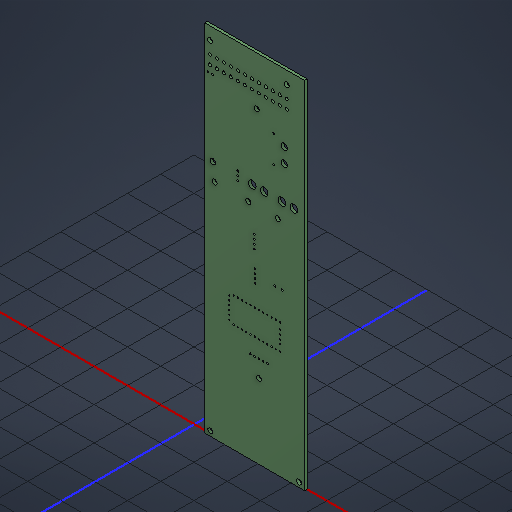
# Autodesk Inventor part: Omnibot_battery_module.brdКонтур
Saved by Autodesk Inventor 2025 (Build 290162000, 162)
## iProperties
Created: 2024-08-15
Part Number: Omnibot_battery_module.brdКонтур
Material: Типовые
Document SubType Name: Modeling
Designer: IvanPetrov
Density: 1 g/cm^3
Appearance: Контур панели
Author: IvanPetrov
Autodesk Inventor part; units mm, degrees
ref_plane "YZ Plane" through (0, 0, 0) normal (1, 0, 0) x (0, 1, 0)
ref_plane "XZ Plane" through (0, 0, 0) normal (0, 1, 0) x (-1, 0, 0)
ref_plane "XY Plane" through (0, 0, 0) normal (0, 0, 1) x (1, 0, 0)
sketch "Эскиз1" plane through (0, 0, 0) normal (0, 0, 1) x (1, 0, 0)
  line L0 (68.1, 149.83) -> (68.1, -63.84)
  line L1 (68.1, -63.84) -> (8.1, -63.84)
  line L2 (8.1, -63.84) -> (8.1, 149.83)
  line L3 (8.1, 149.83) -> (68.1, 149.83)
  circle A0 centre (38.35, 29.21) radius 0.51
  circle A1 centre (38.35, 31.75) radius 0.51
  circle A2 centre (38.35, 34.29) radius 0.51
  circle A3 centre (38.35, 36.83) radius 0.51
  circle A4 centre (37.85, 54.61) radius 0.51
  circle A5 centre (37.85, 52.07) radius 0.51
  circle A6 centre (37.85, 49.53) radius 0.51
  circle A7 centre (37.85, 46.99) radius 0.51
  circle A8 centre (43.86, 79.88) radius 2.275
  circle A9 centre (36.66, 79.88) radius 2.275
  circle A10 centre (61.64, 79.88) radius 2.275
  circle A11 centre (54.44, 79.88) radius 2.275
  circle A12 centre (55.88, 100.33) radius 1.905
  circle A13 centre (55.88, 109.22) radius 1.905
  circle A14 centre (11.19, 134.94) radius 0.9
  circle A15 centre (15.39, 134.94) radius 0.9
  circle A16 centre (19.59, 134.94) radius 0.9
  circle A17 centre (23.79, 134.94) radius 0.9
  circle A18 centre (27.99, 134.94) radius 0.9
  circle A19 centre (32.19, 134.94) radius 0.9
  circle A20 centre (36.39, 134.94) radius 0.9
  circle A21 centre (40.59, 134.94) radius 0.9
  circle A22 centre (44.79, 134.94) radius 0.9
  circle A23 centre (48.99, 134.94) radius 0.9
  circle A24 centre (53.19, 134.94) radius 0.9
  circle A25 centre (57.39, 134.94) radius 0.9
  circle A26 centre (11.19, 129.44) radius 0.9
  circle A27 centre (15.39, 129.44) radius 0.9
  circle A28 centre (19.59, 129.44) radius 0.9
  circle A29 centre (23.79, 129.44) radius 0.9
  circle A30 centre (27.99, 129.44) radius 0.9
  circle A31 centre (32.19, 129.44) radius 0.9
  circle A32 centre (36.39, 129.44) radius 0.9
  circle A33 centre (40.59, 129.44) radius 0.9
  circle A34 centre (44.79, 129.44) radius 0.9
  circle A35 centre (48.99, 129.44) radius 0.9
  circle A36 centre (53.19, 129.44) radius 0.9
  circle A37 centre (57.39, 129.44) radius 0.9
  circle A38 centre (49.53, 113.03) radius 0.51
  circle A39 centre (12.7, 125.35) radius 0.51
  circle A40 centre (10.16, 125.35) radius 0.51
  circle A41 centre (49.53, 96.52) radius 0.51
  circle A42 centre (45.72, -8.89) radius 0.51
  circle A43 centre (43.18, -8.89) radius 0.51
  circle A44 centre (40.64, -8.89) radius 0.51
  circle A45 centre (38.1, -8.89) radius 0.51
  circle A46 centre (35.56, -8.89) radius 0.51
  circle A47 centre (43.18, 16.51) radius 0.4
  circle A48 centre (40.64, 16.51) radius 0.4
  circle A49 centre (38.1, 16.51) radius 0.4
  circle A50 centre (35.56, 16.51) radius 0.4
  circle A51 centre (53.34, 5.08) radius 0.4
  circle A52 centre (53.34, 7.62) radius 0.4
  circle A53 centre (53.34, 10.16) radius 0.4
  circle A54 centre (53.34, 12.7) radius 0.4
  circle A55 centre (35.56, 1.27) radius 0.4
  circle A56 centre (38.1, 1.27) radius 0.4
  circle A57 centre (40.64, 1.27) radius 0.4
  circle A58 centre (43.18, 1.27) radius 0.4
  circle A59 centre (45.72, 1.27) radius 0.4
  circle A60 centre (48.26, 1.27) radius 0.4
  circle A61 centre (50.8, 1.27) radius 0.4
  circle A62 centre (53.34, 1.27) radius 0.4
  circle A63 centre (53.34, 16.51) radius 0.4
  circle A64 centre (50.8, 16.51) radius 0.4
  circle A65 centre (48.26, 16.51) radius 0.4
  circle A66 centre (45.72, 16.51) radius 0.4
  circle A67 centre (22.86, 15.24) radius 0.4
  circle A68 centre (27.94, 16.51) radius 0.4
  circle A69 centre (33.02, 1.27) radius 0.4
  circle A70 centre (22.86, 2.54) radius 0.4
  circle A71 centre (22.86, 5.08) radius 0.4
  circle A72 centre (25.4, 16.51) radius 0.4
  circle A73 centre (30.48, 16.51) radius 0.4
  circle A74 centre (30.48, 1.27) radius 0.4
  circle A75 centre (27.94, 1.27) radius 0.4
  circle A76 centre (22.86, 10.16) radius 0.4
  circle A77 centre (25.4, 1.27) radius 0.4
  circle A78 centre (22.86, 12.7) radius 0.4
  circle A79 centre (33.02, 16.51) radius 0.4
  circle A80 centre (22.86, 7.62) radius 0.4
  circle A81 centre (27.94, 80.01) radius 0.51
  circle A82 centre (27.94, 82.55) radius 0.51
  circle A83 centre (27.94, 77.47) radius 0.51
  circle A84 centre (52.07, 69.85) radius 1.5
  circle A85 centre (34.29, 69.85) radius 1.5
  circle A86 centre (13.97, 69.85) radius 1.5
  circle A87 centre (11.43, -60.96) radius 1.5
  circle A88 centre (64.77, -60.96) radius 1.5
  circle A89 centre (40.64, -19.05) radius 1.5
  circle A90 centre (39.37, 120.65) radius 1.5
  circle A91 centre (57.39, 142.24) radius 1.5
  circle A92 centre (11.19, 142.24) radius 1.5
  circle A93 centre (12.954, 80.01) radius 1.651
  circle A94 centre (50.245, 33.8614) radius 0.6
  circle A95 centre (54.61, 33.909) radius 0.6
  constraints: 96 centre point, 8 end point
extrude "Omnibot_battery_module.brdКонтур" add sketch "Эскиз1" along normal blind 1.6
